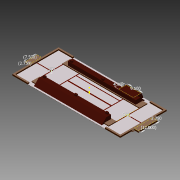
# Autodesk Inventor part: Ball Field
Saved by Autodesk Inventor 2015 (Build 190159000, 159)
## iProperties
Created: 2016-11-29
Part Number: Ball Field
Material: Generic
Document SubType Name: Modeling
Designer: Simms
Density: 1 g/cm^3
Appearance: Default
Author: Simms
Autodesk Inventor part; units mm, degrees
ref_plane "YZ Plane" through (0, 0, 0) normal (1, 0, 0) x (0, 1, 0)
sketch "Sketch1" plane through (0, 0, 0) normal (0, 1, 0) x (-1, 0, 0)
  line L0 (0, 381) -> (-889, 381)
  line L1 (-889, 381) -> (-889, -381)
  line L2 (-889, -381) -> (0, -381)
  line L3 (0, 381) -> (0, -381)
  point P0 (0, 0)
  dimension "d1" = 762
  dimension "d35" = 889
  constraints: 8 end point, 1 horizontal, 1 parallel, 1 perpendicular
  measures "d1" distance of L1.end L0.end
  measures "d35" distance between parallel lines of L1 L3
extrude "Extrusion1" add sketch "Sketch1" along normal blind 2.54
sketch "Sketch2" plane through (0, 2.54, 0) normal (0, 1, 0) x (1, 0, 0)
  line L0 (0, -381) -> (889, -381) projected
  line L1 (889, -381) -> (889, 381) projected
  line L2 (889, 381) -> (0, 381) projected
  line L3 (863.6, -355.6) -> (635, -355.6)
  line L4 (635, 355.6) -> (863.6, 355.6)
  line L5 (863.6, 355.6) -> (863.6, -355.6)
  line L6 (635, -381) -> (635, -355.6)
  line L7 (635, 355.6) -> (635, 381)
  line L8 (0, 381) -> (0, -381) projected
  line L9 (635, -355.6) -> (635, 355.6) construction
  line L10 (622.3, 190.5) -> (622.3, -190.5)
  line L11 (863.6, 6.35) -> (863.6, -6.35)
  line L12 (863.6, -6.35) -> (635, -6.35)
  line L13 (635, -190.5) -> (635, -6.35)
  line L14 (635, 6.35) -> (635, 190.5)
  line L15 (635, 6.35) -> (863.6, 6.35)
  line L16 (0, -190.5) -> (0, -317.5)
  line L17 (0, -317.5) -> (635, -317.5)
  line L18 (635, -317.5) -> (635, -190.5)
  line L19 (622.3, -190.5) -> (0, -190.5)
  line L20 (0, 0) -> (889, 0) construction
  line L21 (0, 190.5) -> (0, 317.5)
  line L22 (0, 317.5) -> (635, 317.5)
  line L23 (635, 317.5) -> (635, 190.5)
  line L24 (622.3, 190.5) -> (0, 190.5)
  line L25 (368.3, 190.5) -> (368.3, -190.5)
  line L26 (622.3, -190.5) -> (635, -190.5)
  line L27 (622.3, 190.5) -> (635, 190.5)
  line L28 (0, 0) -> (1199.5673, 0) construction
  line L29 (355.6, -9.525) -> (0, -9.525)
  line L30 (0, -9.525) -> (0, 9.525)
  line L31 (0, 9.525) -> (355.6, 9.525)
  line L32 (0, 133.35) -> (355.6, 133.35)
  line L33 (0, 146.05) -> (0, 133.35)
  line L34 (355.6, 146.05) -> (0, 146.05)
  line L35 (355.6, 9.525) -> (355.6, 133.35)
  line L36 (355.6, 146.05) -> (355.6, 190.5)
  line L37 (0, -133.35) -> (355.6, -133.35)
  line L38 (0, -146.05) -> (0, -133.35)
  line L39 (355.6, -146.05) -> (0, -146.05)
  line L40 (355.6, -190.5) -> (355.6, -146.05)
  line L41 (355.6, -133.35) -> (355.6, -9.525)
  line L42 (635, -381) -> (889, -381)
  line L43 (889, -381) -> (889, 381)
  line L44 (889, 381) -> (635, 381)
  line L45 (889, 381) -> (0, 381) projected
  point P0 (745.8337, 0)
  point P1 (599.7837, 0)
  point P2 (345.7837, 88.9)
  dimension "d4" = 25.4
  dimension "d5" = 254
  dimension "d8" = 12.7
  dimension "d11" = 127
  dimension "d16" = 19.05
  dimension "d19" = 63.5
  dimension "d21" = 44.45
  dimension "d22" = 12.7
  dimension "d23" = 374.65
  dimension "d36" = 25.4
  dimension "d37" = 0
  dimension "d38" = 0
  dimension "d39" = 0
  dimension "d40" = 0
  dimension "d41" = 254
  dimension "d42" = 12.7
  dimension "d43" = 12.7
  dimension "d44" = 0
  dimension "d45" = 12.7
  dimension "d46" = 0
  dimension "d47" = 12.7
  constraints: 83 end point, 11 parallel, 6 horizontal, 4 point on line, 3 collinear, 3 perpendicular, 2 midpoint, 1 vertical
  measures "d4" distance between parallel lines of L0 L3
  measures "d5" distance from line of L3.end L1
  measures "d8" distance of L10.start L14.end
  measures "d11" distance of L16.end L16.start
  measures "d16" distance of L29.end L30.end
  measures "d19" distance between parallel lines of L17 L0
  measures "d21" distance between parallel lines of L24 L34
  measures "d22" distance between parallel lines of L15 L12
  measures "d23" distance between parallel lines of L12 L0
  measures "d36" distance between parallel lines of L5 L1
  measures "d37" distance between parallel lines of L5 L11
  measures "d38" distance between parallel lines of L18 L9
  measures "d39" distance between parallel lines of L9 L14
  measures "d40" distance between parallel lines of L8 L16
  measures "d41" distance between parallel lines of L10 L25
  measures "d42" distance between parallel lines of L25 L40
  measures "d43" distance between parallel lines of L25 L36
  measures "d44" distance between parallel lines of L8 L30
  measures "d45" distance between parallel lines of L25 L35
  measures "d46" distance between parallel lines of L8 L38
  measures "d47" distance between parallel lines of L25 L41
extrude "Extrusion2" add sketch "Sketch2" along normal blind 12.7 contours L8 L19 L26 L18 L17 | L24 L8 L22 L23 L27
extrude "Extrusion3" add sketch "Sketch2" along normal blind 19.05 contours L6 L3 L5 L4 L7 L2 L1 L0
extrude "Extrusion4" add sketch "Sketch2" along normal blind 0.254 contours L8 L37 L41 L29 L31 L35 L32 L34 L36 L24 L25 L19 L40 L39 | L26 L10 L27 L14 L15 L5 L12 L13
sketch "Sketch3" plane through (0, 0, -381) normal (-1, 0, 0) x (0, 0, 1)
  line L0 (762, 0) -> (0, 0) projected
  line L1 (762, 0) -> (762, 2.54) projected
  line L2 (698.5, 2.54) -> (762, 2.54) projected
  line L3 (698.5, 2.54) -> (698.5, 15.24) projected
  line L4 (571.5, 15.24) -> (698.5, 15.24) projected
  line L5 (571.5, 2.54) -> (571.5, 15.24) projected
  line L6 (527.05, 2.54) -> (571.5, 2.54) projected
  line L7 (527.05, 2.54) -> (527.05, 2.794) projected
  line L8 (514.35, 2.794) -> (527.05, 2.794) projected
  line L9 (514.35, 2.54) -> (514.35, 2.794) projected
  line L10 (390.525, 2.54) -> (514.35, 2.54) projected
  line L11 (390.525, 2.54) -> (390.525, 2.794) projected
  line L12 (371.475, 2.794) -> (390.525, 2.794) projected
  line L13 (371.475, 2.54) -> (371.475, 2.794) projected
  line L14 (247.65, 2.54) -> (371.475, 2.54) projected
  line L15 (247.65, 2.54) -> (247.65, 2.794) projected
  line L16 (234.95, 2.794) -> (247.65, 2.794) projected
  line L17 (234.95, 2.54) -> (234.95, 2.794) projected
  line L18 (190.5, 2.54) -> (234.95, 2.54) projected
  line L19 (190.5, 2.54) -> (190.5, 15.24) projected
  line L20 (63.5, 15.24) -> (190.5, 15.24) projected
  line L21 (63.5, 2.54) -> (63.5, 15.24) projected
  line L22 (0, 2.54) -> (63.5, 2.54) projected
  line L23 (0, 0) -> (0, 2.54) projected
  line L24 (736.6, 2.54) -> (584.2, 2.54)
  line L25 (387.35, 2.54) -> (698.5, 2.54) projected
  line L26 (736.6, 2.54) -> (889, 2.54) construction
  line L27 (736.6, 2.54) -> (660.4, 78.74)
  line L28 (736.6, 2.54) -> (844.3631, 2.54) construction
  line L29 (660.4, 78.74) -> (584.2, 78.74)
  line L30 (762, 0) -> (0, 0) projected
  line L31 (584.2, 78.74) -> (584.2, 2.54)
  line L32 (381, 2.54) -> (381, -13.3549) construction
  line L33 (25.4, 2.54) -> (177.8, 2.54)
  line L34 (374.65, 2.54) -> (63.5, 2.54)
  line L35 (25.4, 2.54) -> (101.6, 78.74)
  line L36 (101.6, 78.74) -> (177.8, 78.74)
  line L37 (177.8, 78.74) -> (177.8, 2.54)
  point P0 (381, 0)
  dimension "d30" = 152.4
  dimension "d31" = 180
  dimension "d32" = 135
  constraints: 24 end point, 5 symmetric about line, 2 equal length, 2 horizontal, 1 collinear, 1 parallel, 1 perpendicular, 1 vertical
  measures "d30" distance of L24.start L24.end
  measures "d31" angle of L24 L26
  measures "d32" angle of L28 L27
extrude "Extrusion5" add sketch "Sketch3" against normal blind 558.8 contours L2 L3 L4 L31 L29 L27 | L35 L36 L37 L20 L21 L22 | L24 L31 L4 L3 | L21 L20 L37 L33
mirror "Mirror1" about plane through (0, 0, 0) normal (1, 0, 0) of "Extrusion1", "Extrusion2", "Extrusion3", "Extrusion4", "Extrusion5"
sketch "Sketch4" plane through (558.8, 78.74, 279.4) normal (0, 1, 0) x (1, 0, 0)
  line L0 (-203.2, 133.35) -> (-914.4, 133.35) construction
  line L1 (-203.2, 133.35) -> (-203.2, 88.9) construction
  line L2 (-190.5, 88.9) -> (-203.2, 88.9) construction
  line L3 (-190.5, 88.9) -> (-190.5, 469.9) construction
  line L4 (-203.2, 469.9) -> (-190.5, 469.9) construction
  line L5 (-203.2, 469.9) -> (-203.2, 425.45) construction
  line L6 (-203.2, 425.45) -> (-914.4, 425.45) construction
  line L7 (-914.4, 469.9) -> (-914.4, 425.45) construction
  line L8 (-914.4, 469.9) -> (-927.1, 469.9) construction
  line L9 (-927.1, 88.9) -> (-927.1, 469.9) construction
  line L10 (-927.1, 88.9) -> (-914.4, 88.9) construction
  line L11 (-914.4, 133.35) -> (-914.4, 88.9) construction
  line L12 (-203.2, 146.05) -> (-914.4, 146.05) construction
  line L13 (-914.4, 269.875) -> (-914.4, 146.05) construction
  line L14 (-203.2, 269.875) -> (-914.4, 269.875) construction
  line L15 (-203.2, 269.875) -> (-203.2, 146.05) construction
  line L16 (-203.2, 288.925) -> (-914.4, 288.925) construction
  line L17 (-914.4, 412.75) -> (-914.4, 288.925) construction
  line L18 (-203.2, 412.75) -> (-914.4, 412.75) construction
  line L19 (-203.2, 412.75) -> (-203.2, 288.925) construction
  line L20 (-25.4, 69.85) -> (-63.5, 69.85)
  line L21 (-63.5, 69.85) -> (-63.5, 44.45)
  line L22 (-63.5, 44.45) -> (-25.4, 44.45)
  line L23 (-25.4, 44.45) -> (-25.4, 69.85)
  line L24 (0, 76.2) -> (-1117.6, 76.2) construction
  line L25 (0, 76.2) -> (0, -38.1) construction
  line L26 (-539.75, 69.85) -> (-558.8, 69.85)
  line L27 (-558.8, 44.45) -> (-539.75, 44.45)
  line L28 (-539.75, 44.45) -> (-539.75, 69.85)
  line L29 (-1092.2, 69.85) -> (-1054.1, 69.85)
  line L30 (-1054.1, 69.85) -> (-1054.1, 44.45)
  line L31 (-1054.1, 44.45) -> (-1092.2, 44.45)
  line L32 (-1092.2, 44.45) -> (-1092.2, 69.85)
  line L33 (-577.85, 69.85) -> (-558.8, 69.85)
  line L34 (-558.8, 44.45) -> (-577.85, 44.45)
  line L35 (-577.85, 44.45) -> (-577.85, 69.85)
  line L36 (-558.8, 279.4) -> (-687.566, 279.4) construction
  line L37 (-558.8, 279.4) -> (-430.034, 279.4) construction
  line L38 (-539.75, 488.95) -> (-558.8, 488.95)
  line L39 (-558.8, 514.35) -> (-539.75, 514.35)
  line L40 (-539.75, 514.35) -> (-539.75, 488.95)
  line L41 (-577.85, 488.95) -> (-558.8, 488.95)
  line L42 (-577.85, 514.35) -> (-577.85, 488.95)
  line L43 (-558.8, 514.35) -> (-577.85, 514.35)
  line L44 (-1092.2, 488.95) -> (-1054.1, 488.95)
  line L45 (-1054.1, 488.95) -> (-1054.1, 514.35)
  line L46 (-1054.1, 514.35) -> (-1092.2, 514.35)
  line L47 (-1092.2, 514.35) -> (-1092.2, 488.95)
  dimension "d48" = 38.1
  dimension "d49" = 25.4
  dimension "d50" = 6.35
  dimension "d51" = 25.4
  dimension "d52" = 19.05
  dimension "d53" = 25.4
  dimension "d55" = 180
  constraints: 52 end point, 10 symmetric about line, 3 horizontal, 3 parallel, 3 point on line, 1 collinear, 1 perpendicular
  measures "d48" distance of L22.end L21.end
  measures "d49" distance of L21.end L20.end
  measures "d50" distance between parallel lines of L20 L24
  measures "d51" distance between parallel lines of L25 L23
  measures "d52" distance of L27.end L27.start
  measures "d53" distance of L27.start L26.end
  measures "d55" angle of L36 L37
extrude "Extrusion6" add sketch "Sketch4" along normal blind 25.4
sketch "Sketch5" plane through (495.3, 78.74, 234.95) normal (0, 0, 1) x (1, 0, 0)
  line L0 (63.5, 0) -> (-1054.1, 0) projected
  line L1 (15.875, 0) -> (22.225, 0)
  line L2 (22.225, 0) -> (22.225, 19.05)
  line L3 (22.225, 19.05) -> (15.875, 19.05)
  line L4 (15.875, 19.05) -> (15.875, 0)
  line L5 (0, 0) -> (0, 25.4) projected
  line L6 (0, 0) -> (3.175, 0)
  line L7 (3.175, 0) -> (3.175, 19.05)
  line L8 (3.175, 19.05) -> (0, 19.05)
  line L9 (0, 19.05) -> (0, 0)
  line L10 (38.1, 0) -> (34.925, 0)
  line L11 (34.925, 0) -> (34.925, 19.05)
  line L12 (34.925, 19.05) -> (38.1, 19.05)
  line L13 (38.1, 19.05) -> (38.1, 0)
  point P0 (-495.3, -78.74)
  dimension "d58" = 6.35
  dimension "d59" = 19.05
  dimension "d60" = 15.875
  dimension "d61" = 3.175
  dimension "d62" = 3.175
  constraints: 24 end point, 6 parallel, 3 horizontal, 3 perpendicular, 1 point on line
  measures "d58" distance of L3.end L2.end
  measures "d59" distance of L2.end L1.end
  measures "d60" distance between parallel lines of L4 L5
  measures "d61" distance of L8.end L7.end
  measures "d62" distance of L11.end L12.end
extrude "Extrusion7" cut sketch "Sketch5" against normal blind 25.4
pattern_linear "Rectangular Pattern1" count 3 spacing 514.35 along (-1, 0, 0) count 2 spacing 444.5 along (0, 0, -1) of "Extrusion7"
sketch "Sketch6" plane through (0, 21.59, 0) normal (0, 1, 0) x (1, 0, 0)
  line L0 (889, -381) -> (889, 381) projected
  line L1 (889, 381) -> (635, 381) projected
  line L2 (635, 381) -> (635, 355.6) projected
  line L3 (635, 355.6) -> (863.6, 355.6) projected
  line L4 (863.6, 355.6) -> (863.6, -355.6) projected
  line L5 (863.6, -355.6) -> (635, -355.6) projected
  line L6 (635, -355.6) -> (635, -381) projected
  line L7 (635, -381) -> (889, -381) projected
  line L8 (-558.8, -203.2) -> (558.8, -203.2) projected
  line L9 (558.8, -203.2) -> (558.8, -317.5) projected
  line L10 (558.8, -317.5) -> (635, -317.5) projected
  line L11 (635, -317.5) -> (635, -190.5) projected
  line L12 (635, -190.5) -> (-635, -190.5) projected
  line L13 (-635, -317.5) -> (-635, -190.5) projected
  line L14 (-558.8, -317.5) -> (-635, -317.5) projected
  line L15 (-558.8, -203.2) -> (-558.8, -317.5) projected
  line L16 (558.8, 317.5) -> (558.8, 203.2) projected
  line L17 (-558.8, 203.2) -> (558.8, 203.2) projected
  line L18 (-558.8, 317.5) -> (-558.8, 203.2) projected
  line L19 (-635, 317.5) -> (-558.8, 317.5) projected
  line L20 (-635, 190.5) -> (-635, 317.5) projected
  line L21 (635, 190.5) -> (-635, 190.5) projected
  line L22 (635, 190.5) -> (635, 317.5) projected
  line L23 (635, 317.5) -> (558.8, 317.5) projected
  line L24 (889, -381) -> (889, 381) projected
  line L25 (889, -196.85) -> (965.2, -196.85)
  line L26 (965.2, -196.85) -> (965.2, 196.85)
  line L27 (965.2, 196.85) -> (889, 196.85)
  line L28 (889, 196.85) -> (889, -196.85)
  line L29 (-889, 381) -> (-889, -381) projected
  line L30 (-889, 0) -> (-965.2, 0) construction
  line L31 (-965.2, 0) -> (-965.2, 101.6)
  line L32 (-965.2, 101.6) -> (-889, 101.6)
  line L33 (-889, 101.6) -> (-889, 0)
  line L34 (-965.2, 0) -> (-965.2, -101.6)
  line L35 (-965.2, -101.6) -> (-889, -101.6)
  line L36 (-889, -101.6) -> (-889, 0)
  point P0 (0, 0)
  dimension "d71" = 76.2
  dimension "d72" = 393.7
  dimension "d73" = 76.2
  dimension "d74" = 101.6
  dimension "d80" = 184.15
  constraints: 22 end point, 4 parallel, 2 horizontal, 2 perpendicular, 2 symmetric about line, 1 midpoint, 1 point on line
  measures "d71" distance of L27.end L26.end
  measures "d72" distance of L26.end L25.end
  measures "d73" distance of L31.end L32.end
  measures "d74" distance of L30.end L31.end
  measures "d80" distance between parallel lines of L25 L7
extrude "Extrusion8" add sketch "Sketch6" against normal up to surface (21.59 mm away) from surface at 0 contours L0 L27 L26 L25 | L29 L35 L34 L31 L32
sketch "Sketch7" plane through (889, 21.59, 196.85) normal (0, 0, 1) x (1, 0, 0)
  line L0 (0, 0) -> (21.59, -21.59)
  line L1 (0, 0) -> (30.5329, 0) construction
  line L2 (0, 0) -> (76.2, 0)
  line L3 (76.2, 0) -> (0, 0) projected
  line L4 (76.2, 0) -> (76.2, -21.59)
  line L5 (76.2, -21.59) -> (21.59, -21.59)
  point P0 (-889, -21.59)
  dimension "d77" = 45
  constraints: 10 end point, 2 perpendicular, 1 collinear, 1 equal length, 1 horizontal
  measures "d77" angle of L0 L1
extrude "Extrusion9" cut sketch "Sketch7" against normal blind 38.1
ref_plane "Work Plane1" through (889, 0, 0) normal (0, 0, 1) x (1, 0, 0)
mirror "Mirror2" about plane through (889, 0, 0) normal (0, 0, 1) of "Extrusion9"
ref_plane "Work Plane2" through (508, 0, -381) normal (1, 0, 0) x (0, 0, -1)
sketch "Sketch8" plane through (508, 0, -381) normal (1, 0, 0) x (0, 0, -1)
  line L0 (-25.4, 2.54) -> (-63.5, 2.54) projected
  line L1 (-63.5, 2.54) -> (-374.65, 2.54) projected
  line L2 (-374.65, 2.54) -> (-25.4, 2.54) projected
  line L3 (-25.4, 2.54) -> (0, 2.54) projected
  line L4 (-25.4, 2.54) -> (0, 2.54) projected
  line L5 (-374.65, 2.54) -> (-25.4, 2.54) projected
  line L6 (-63.5, 2.54) -> (-374.65, 2.54) projected
  line L7 (-25.4, 2.54) -> (-63.5, 2.54) projected
  line L8 (-63.5, 2.54) -> (-63.5, 15.24) projected
  line L9 (-25.4, 2.54) -> (-63.5, 2.54) projected
  line L10 (-25.4, 2.54) -> (-101.6, 78.74) projected
  line L11 (-101.6, 78.74) -> (-177.8, 78.74) projected
  line L12 (-177.8, 78.74) -> (-177.8, 15.24) projected
  line L13 (-63.5, 15.24) -> (-177.8, 15.24) projected
  line L14 (0, 2.54) -> (-27.7345, 78.74)
  line L15 (0, 2.54) -> (81.0903, 2.54) construction
  line L16 (-27.7345, 78.74) -> (-101.6, 78.74)
  line L17 (-101.6, 78.74) -> (-101.6, 2.54)
  line L18 (0, 2.54) -> (-101.6, 2.54)
  point P0 (-381, 0)
  dimension "d82" = 110
  constraints: 10 end point, 2 horizontal, 2 perpendicular, 1 equal length, 1 point on line
  measures "d82" angle of L15 L14
extrude "Extrusion10" add sketch "Sketch8" against normal blind 254 contours L10 L16 L14 L3 | L0 L8 L13 L17 L10 | L1 L17 L13 L8
sketch "Sketch9" plane through (0, 21.59, 0) normal (0, 1, 0) x (1, 0, 0)
  line L0 (889, -152.4) -> (958.85, -152.4) construction
  line L1 (958.85, -152.4) -> (958.85, 152.4) construction
  line L2 (958.85, 152.4) -> (889, 152.4) construction
  line L3 (889, 152.4) -> (889, -152.4) construction
  line L4 (-958.85, -95.25) -> (-889, -95.25) construction
  line L5 (-889, -95.25) -> (-889, 95.25) construction
  line L6 (-889, 95.25) -> (-958.85, 95.25) construction
  line L7 (-958.85, 95.25) -> (-958.85, -95.25) construction
  point P0 (0, 0)
  dimension "d88" = 304.8
  dimension "d89" = 69.85
  dimension "d94" = 190.5
  dimension "d95" = 69.85
  constraints: 16 end point, 4 parallel, 2 horizontal, 2 perpendicular
  measures "d88" distance of L0.end L1.end
  measures "d89" distance of L1.end L2.end
  measures "d94" distance of L6.end L4.start
  measures "d95" distance of L4.start L4.end
sketch "Sketch10" plane through (558.8, 78.74, -203.2) normal (0, 1, 0) x (1, 0, 0)
  line L0 (-298.45, 143.7155) -> (-57.15, 143.7155) construction
  line L1 (-57.15, 143.7155) -> (-57.15, 19.05) construction
  line L2 (-57.15, 19.05) -> (-298.45, 19.05) construction
  line L3 (-298.45, 19.05) -> (-298.45, 143.7155) construction
  point P0 (-558.8, -203.2)
  dimension "d100" = 124.6655
  dimension "d101" = 241.3
  constraints: 8 end point, 2 parallel, 1 horizontal, 1 perpendicular
  measures "d100" distance of L2.end L0.start
  measures "d101" distance of L0.start L0.end
sketch "Sketch11" plane through (558.8, 15.24, -203.2) normal (0, 0, 1) x (1, 0, 0)
  line L0 (-561.975, 57.15) -> (-555.625, 57.15) construction
  line L1 (-555.625, 57.15) -> (-555.625, 44.45) construction
  line L2 (-555.625, 44.45) -> (-561.975, 44.45) construction
  line L3 (-561.975, 44.45) -> (-561.975, 57.15) construction
  line L4 (-1117.6, 63.5) -> (0, 63.5) projected
  line L5 (-1117.6, 63.5) -> (-1117.6, 0) projected
  point P0 (-558.8, -15.24)
  dimension "d102" = 6.35
  dimension "d103" = 12.7
  dimension "d108" = 6.35
  dimension "d109" = 555.625
  constraints: 8 end point, 2 parallel, 1 horizontal, 1 perpendicular
  measures "d102" distance of L0.start L0.end
  measures "d103" distance between parallel lines of L2 L0
  measures "d108" distance between parallel lines of L0 L4
  measures "d109" distance between parallel lines of L5 L3
sketch "Sketch12" plane through (558.8, 15.24, 203.2) normal (0, 0, -1) x (-1, 0, 0)
  line L0 (561.975, 44.45) -> (561.975, 57.15) construction
  line L1 (561.975, 57.15) -> (555.625, 57.15) construction
  line L2 (555.625, 57.15) -> (555.625, 44.45) construction
  line L3 (555.625, 44.45) -> (561.975, 44.45) construction
  point P0 (558.8, -15.24)
sketch "Sketch13" plane through (0, 2.794, 0) normal (0, 1, 0) x (1, 0, 0)
  line L0 (622.3, -190.5) -> (622.3, 190.5) construction
  line L1 (635, -6.35) -> (652.9605, -6.35) construction
  circle A0 centre (628.65, 0) radius 6.35 construction
  circle A1 centre (-628.65, 0) radius 6.35 construction
  point P0 (0, 0)
  dimension "d106" = 12.7
  dimension "d107" = 12.7
  constraints: 2 centre point, 2 end point, 1 horizontal
  measures "d106" diameter of A1
  measures "d107" diameter of A0
body "Solid1"
